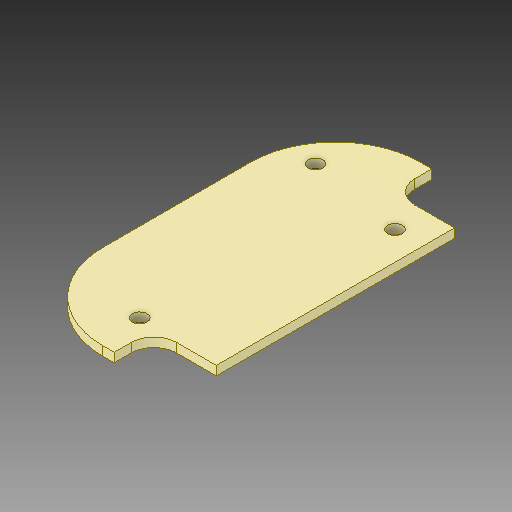
# Autodesk Inventor part: PCB Gauche
Saved by Autodesk Inventor 2019 (Build 230136000, 136)
## iProperties
Created: 2018-06-08
Part Number: PCB Gauche
Material: Nylon, disulfure de molybdène
Document SubType Name: Modeling
Designer: dimercur
Density: 1.13 g/cm^3
Appearance: Nylon 6
Mass: 2.24944 g
Surface Area: 27.2645 cm^2
Volume: 1.99065 cm^3
Author: dimercur
Autodesk Inventor part; units mm, degrees
ref_plane "YZ Plane" through (0, 0, 0) normal (1, 0, 0) x (0, 1, 0)
ref_plane "XZ Plane" through (0, 0, 0) normal (0, 1, 0) x (-1, 0, 0)
ref_plane "XY Plane" through (0, 0, 0) normal (0, 0, 1) x (1, 0, 0)
sketch "Esquisse1" plane through (0, 0, 0) normal (0, 1, 0) x (-1, 0, 0)
  line L0 (14, -28) -> (-14, -28)
  line L1 (-14, -28) -> (-14, 28)
  line L2 (-14, 28) -> (14, 28)
  line L3 (14, 28) -> (14, -28)
  point P0 (0, 0)
  dimension "d0" = 28
  dimension "d1" = 56
  dimension "d2" = 28
  dimension "d3" = 14
  constraints: 8 end point, 2 parallel, 1 horizontal, 1 perpendicular
  measures "d0" distance of L0.start L0.end
  measures "d1" distance of L2.end L0.start
  measures "d2" vertical distance of point (0, 0) L0.start
  measures "d3" horizontal distance of point (0, 0) L0.start
extrude "Extrusion1" add sketch "Esquisse1" along normal blind 1.6
fillet "Congé1" radius 15 2 edges at (-14, 0.8, -28) (-14, 0.8, 28)
sketch "Esquisse2" plane through (0, 1.6, 0) normal (0, 1, 0) x (1, 0, 0)
  circle A0 centre (7, 25) radius 4
  circle A1 centre (7, -25) radius 4
  line L0 (1, -28) -> (14, -28) projected
  line L1 (3, 25) -> (3, 28)
  line L2 (14, 28) -> (1, 28) projected
  line L3 (4.3542, 28) -> (3, 28)
  line L4 (9.6458, 28) -> (14, 28)
  line L5 (14, 28) -> (14, 21)
  line L6 (14, -28) -> (14, 28) projected
  line L7 (14, 21) -> (7, 21)
  line L8 (7, -21) -> (14, -21)
  line L9 (14, -21) -> (14, -28)
  line L10 (14, -28) -> (9.6458, -28)
  line L11 (3, -25) -> (3, -28)
  line L12 (3, -28) -> (4.3542, -28)
  point P0 (0, 0)
  dimension "d7" = 8
  dimension "d8" = 7
  dimension "d9" = 7
  dimension "d10" = 25
  dimension "d11" = 25
  constraints: 20 end point, 10 point on line, 8 point on circle, 2 centre point, 2 collinear, 2 tangent, 1 equal radius, 1 parallel, 1 perpendicular, 1 vertical
  measures "d7" diameter of A0
  measures "d8" horizontal distance of point (0, 0) A0.centre
  measures "d9" horizontal distance of point (0, 0) A1.centre
  measures "d10" vertical distance of point (0, 0) A0.centre
  measures "d11" vertical distance of point (0, 0) A1.centre
extrude "Extrusion3" cut sketch "Esquisse2" against normal through all contours A0 L2 | A0 L2 L5 L7 | A0 L1 L2 | A1 L0 | A1 L8 L6 L0 | A1 L0 L11 picked at (8.3035, 24.6872) picked at (8.2117, -25.5325)
sketch "Esquisse3" plane through (0, 1.6, 0) normal (0, 1, 0) x (1, 0, 0)
  circle A0 centre (-8, 18.5) radius 1.3
  circle A1 centre (0, -20.5) radius 1.3
  circle A2 centre (9, 15.5) radius 1.3
  line L0 (-14, 13) -> (-14, -13) projected
  point P0 (0, 0)
  dimension "d19" = 2.6
  dimension "d20" = 2.6
  dimension "d21" = 2.6
  dimension "d22" = 20.5
  dimension "d23" = 14
  dimension "d24" = 18.5
  dimension "d25" = 6
  dimension "d26" = 15.5
  dimension "d27" = 9
  constraints: 3 centre point
  measures "d19" diameter of A0
  measures "d20" diameter of A2
  measures "d21" diameter of A1
  measures "d22" distance of A1.centre point (0, 0)
  measures "d23" distance from line of L0 A1.centre
  measures "d24" vertical distance of point (0, 0) A0.centre
  measures "d25" distance from line of L0 A0.centre
  measures "d26" vertical distance of point (0, 0) A2.centre
  measures "d27" horizontal distance of point (0, 0) A2.centre
extrude "Extrusion4" cut sketch "Esquisse3" against normal through all
equation "\"d2\" = 0.5 * d1"
equation "\"d3\" = 0.5 * d0"
equation "\"d9\" = d8"
equation "\"d11\" = d10"
equation "\"d20\" = d19"
equation "\"d21\" = d19"
